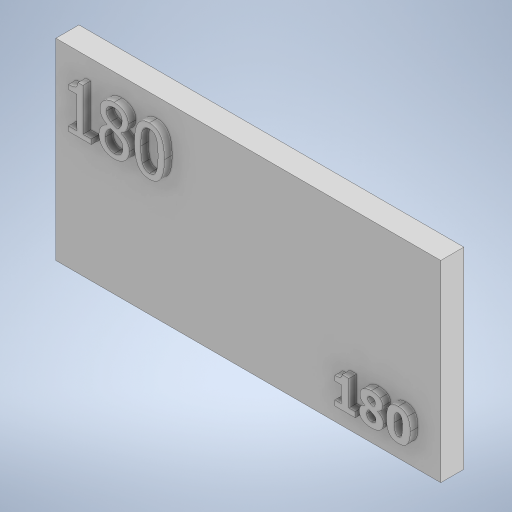
# Autodesk Inventor part: температурный тест
Saved by Autodesk Inventor 2023.1 (Build 271208000, 208)
## iProperties
Created: 2023-03-01
Part Number: температурный тест
Material: Типовые
Document SubType Name: Modeling
Designer: User
Density: 1 g/cm^3
Appearance: По умолчанию
Author: User
Autodesk Inventor part; units mm, degrees
ref_plane "YZ Plane" through (0, 0, 0) normal (1, 0, 0) x (0, 1, 0)
ref_plane "XZ Plane" through (0, 0, 0) normal (0, 1, 0) x (-1, 0, 0)
ref_plane "XY Plane" through (0, 0, 0) normal (0, 0, 1) x (1, 0, 0)
sketch "Эскиз1" plane through (0, 0, 0) normal (0, 0, 1) x (1, 0, 0)
  line L0 (-25, 12.5) -> (25, 12.5)
  line L1 (25, 12.5) -> (25, -12.5)
  line L2 (25, -12.5) -> (-25, -12.5)
  line L3 (-25, -12.5) -> (-25, 12.5)
  line L4 (0, -17.5) -> (0, 17.5) projected
  line L5 (-35, 0) -> (35, 0) projected
  line L6 (-15, 7.5) -> (15, 7.5)
  line L7 (15, 7.5) -> (15, -7.5)
  line L8 (15, -7.5) -> (-15, -7.5)
  line L9 (-15, -7.5) -> (-15, 7.5)
  point P0 (0, 0)
  dimension "d0" = 50
  dimension "d1" = 25
  dimension "d2" = 5
  dimension "d3" = 10
  constraints: 16 end point, 4 parallel, 2 horizontal, 2 perpendicular, 4 other
  measures "d0" distance between parallel lines of L1 L3
  measures "d1" distance between parallel lines of L0 L2
  measures "d2" distance between parallel lines of L0 L6
  measures "d3" distance between parallel lines of L1 L7
extrude "Выдавливание1" add sketch "Эскиз1" along normal blind 2 contours L0 L4 L6 L9 L5 L3 | L0 L1 L5 L7 L6 L4 | L5 L9 L8 L4 L2 L3 | L1 L2 L4 L8 L7 L5
sketch "Эскиз2" plane through (0, 0, 2) normal (0, 0, 1) x (1, 0, 0)
  line L0 (-25, 12.5) -> (-25, -12.5) projected
  line L1 (-25, -12.5) -> (25, -12.5) projected
  line L2 (25, -12.5) -> (25, 12.5) projected
  line L3 (25, 12.5) -> (-25, 12.5) projected
  line L4 (-15, 7.5) -> (15, 7.5) projected
  line L5 (15, 7.5) -> (15, -7.5) projected
  line L6 (15, -7.5) -> (-15, -7.5) projected
  line L7 (-15, -7.5) -> (-15, 7.5) projected
  point P0 (0, 0)
extrude "Выдавливание2" add sketch "Эскиз2" along normal blind 1 contours L3 L2 L1 L0 | L4 L5 L6 L7
sketch "Эскиз3" plane through (0, 0, 3) normal (0, 0, 1) x (1, 0, 0)
  line L0 (-23.2901, 10.0825) -> (-16.4284, 10.0825) construction
  line L1 (-16.4284, 10.0825) -> (-16.4284, 6.8962) construction
  line L2 (-16.4284, 6.8962) -> (-23.2901, 6.8962) construction
  line L3 (-23.2901, 6.8962) -> (-23.2901, 10.0825) construction
  line L4 (11.7335, -5.6604) -> (22.2456, -5.6604) construction
  line L5 (22.2456, -5.6604) -> (22.2456, -9.8451) construction
  line L6 (22.2456, -9.8451) -> (11.7335, -9.8451) construction
  line L7 (11.7335, -9.8451) -> (11.7335, -5.6604) construction
  line L8 (-19.3899, 3.8441) -> (-22.3657, 3.8441)
  line L9 (-22.3657, 3.8441) -> (-22.3657, 4.467)
  line L10 (-22.3657, 4.467) -> (-21.2584, 4.467)
  line L11 (-21.2584, 4.467) -> (-21.2584, 8.5551)
  line L12 (-21.2584, 8.5551) -> (-22.3657, 8.5551)
  line L13 (-22.3657, 8.5551) -> (-22.3657, 9.1137)
  spline S0 degree 2 poles (-22.3657, 9.1137) (-21.7379, 9.1137) (-21.1447, 9.4696) (-21.1052, 9.9639) knots 0 0 0 1 2 2 2
  line L14 (-21.1052, 9.9639) -> (-20.4724, 9.9639)
  line L15 (-20.4724, 9.9639) -> (-20.4724, 4.467)
  line L16 (-20.4724, 4.467) -> (-19.3899, 4.467)
  line L17 (-19.3899, 4.467) -> (-19.3899, 3.8441)
  spline S1 degree 2 poles (-16.4239, 3.7057) (-16.8787, 3.7057) (-17.6251, 3.9776) (-17.8871, 4.2297) knots 0 0 0 1 2 2 2
  spline S2 degree 2 poles (-17.8871, 4.2297) (-18.1441, 4.4769) (-18.4111, 5.1492) (-18.4111, 5.5298) knots 0 0 0 1 2 2 2
  spline S3 degree 2 poles (-18.4111, 5.5298) (-18.4111, 6.0241) (-17.8822, 6.8546) (-17.3779, 7.1018) knots 0 0 0 1 2 2 2
  line L18 (-17.3779, 7.1018) -> (-17.3779, 7.1265)
  spline S4 degree 2 poles (-17.3779, 7.1265) (-17.8278, 7.3885) (-18.2628, 8.0113) (-18.2628, 8.476) knots 0 0 0 1 2 2 2
  spline S5 degree 2 poles (-18.2628, 8.476) (-18.2628, 9.1631) (-17.2247, 10.0825) (-16.4239, 10.0825) knots 0 0 0 1 2 2 2
  spline S6 degree 2 poles (-16.4239, 10.0825) (-15.5934, 10.0825) (-14.5899, 9.2125) (-14.5899, 8.5304) knots 0 0 0 1 2 2 2
  spline S7 degree 2 poles (-14.5899, 8.5304) (-14.5899, 8.1201) (-15.0694, 7.3193) (-15.5193, 7.0919) knots 0 0 0 1 2 2 2
  line L19 (-15.5193, 7.0919) -> (-15.5193, 7.0672)
  spline S8 degree 2 poles (-15.5193, 7.0672) (-14.9854, 6.82) (-14.4367, 6.1082) (-14.4367, 5.5446) knots 0 0 0 1 2 2 2
  spline S9 degree 2 poles (-14.4367, 5.5446) (-14.4367, 4.7636) (-15.5736, 3.7057) (-16.4239, 3.7057) knots 0 0 0 1 2 2 2
  spline S10 degree 2 poles (-15.277, 5.4655) (-15.277, 5.8412) (-15.5736, 6.2861) (-15.9938, 6.5135) knots 0 0 0 1 2 2 2
  spline S11 degree 2 poles (-15.9938, 6.5135) (-16.1322, 6.5926) (-16.5969, 6.7755) (-16.8886, 6.8941) knots 0 0 0 1 2 2 2
  spline S12 degree 2 poles (-16.8886, 6.8941) (-17.2247, 6.6717) (-17.5856, 6.0093) (-17.5856, 5.5891) knots 0 0 0 1 2 2 2
  spline S13 degree 2 poles (-17.5856, 5.5891) (-17.5856, 5.0355) (-16.9182, 4.3137) (-16.414, 4.3137) knots 0 0 0 1 2 2 2
  spline S14 degree 2 poles (-16.414, 4.3137) (-15.8999, 4.3137) (-15.277, 4.9317) (-15.277, 5.4655) knots 0 0 0 1 2 2 2
  spline S15 degree 2 poles (-15.3907, 8.5205) (-15.3907, 8.9308) (-15.9394, 9.4795) (-16.4288, 9.4795) knots 0 0 0 1 2 2 2
  spline S16 degree 2 poles (-16.4288, 9.4795) (-16.8737, 9.4795) (-17.4422, 8.9901) (-17.4422, 8.5699) knots 0 0 0 1 2 2 2
  spline S17 degree 2 poles (-17.4422, 8.5699) (-17.4422, 8.2684) (-17.1505, 7.8482) (-16.8589, 7.6801) knots 0 0 0 1 2 2 2
  spline S18 degree 2 poles (-16.8589, 7.6801) (-16.7353, 7.6109) (-16.2113, 7.3687) (-15.9988, 7.2995) knots 0 0 0 1 2 2 2
  spline S19 degree 2 poles (-15.9988, 7.2995) (-15.6428, 7.5714) (-15.3907, 8.1497) (-15.3907, 8.5205) knots 0 0 0 1 2 2 2
  spline S20 degree 2 poles (-9.8938, 6.8941) (-9.8938, 5.253) (-10.8479, 3.7156) (-11.8415, 3.7156) knots 0 0 0 1 2 2 2
  spline S21 degree 2 poles (-11.8415, 3.7156) (-12.8499, 3.7156) (-13.7941, 5.2826) (-13.7941, 6.8892) knots 0 0 0 1 2 2 2
  spline S22 degree 2 poles (-13.7941, 6.8892) (-13.7941, 8.5402) (-12.84, 10.0677) (-11.8415, 10.0677) knots 0 0 0 1 2 2 2
  spline S23 degree 2 poles (-11.8415, 10.0677) (-10.838, 10.0677) (-9.8938, 8.4859) (-9.8938, 6.8941) knots 0 0 0 1 2 2 2
  spline S24 degree 2 poles (-10.9418, 5.0355) (-10.8232, 5.337) (-10.7243, 6.2663) (-10.7243, 6.8941) knots 0 0 0 1 2 2 2
  spline S25 degree 2 poles (-10.7243, 6.8941) (-10.7243, 7.5219) (-10.8232, 8.4463) (-10.9467, 8.7577) knots 0 0 0 1 2 2 2
  spline S26 degree 2 poles (-10.9467, 8.7577) (-11.0703, 9.0692) (-11.5004, 9.3905) (-11.8415, 9.3905) knots 0 0 0 1 2 2 2
  spline S27 degree 2 poles (-11.8415, 9.3905) (-12.1826, 9.3905) (-12.6225, 9.0692) (-12.751, 8.7479) knots 0 0 0 1 2 2 2
  spline S28 degree 2 poles (-12.751, 8.7479) (-12.8746, 8.4364) (-12.9636, 7.4873) (-12.9636, 6.8892) knots 0 0 0 1 2 2 2
  spline S29 degree 2 poles (-12.9636, 6.8892) (-12.9636, 6.2466) (-12.8845, 5.3864) (-12.756, 5.0503) knots 0 0 0 1 2 2 2
  spline S30 degree 2 poles (-12.756, 5.0503) (-12.6373, 4.7339) (-12.1974, 4.3928) (-11.8415, 4.3928) knots 0 0 0 1 2 2 2
  spline S31 degree 2 poles (-11.8415, 4.3928) (-11.5053, 4.3928) (-11.0654, 4.7142) (-10.9418, 5.0355) knots 0 0 0 1 2 2 2
  line L20 (14.9004, -9.7511) -> (12.2586, -9.7511)
  line L21 (12.2586, -9.7511) -> (12.2586, -9.0542)
  line L22 (12.2586, -9.0542) -> (13.1014, -9.0542)
  line L23 (13.1014, -9.0542) -> (13.1014, -6.9375)
  line L24 (13.1014, -6.9375) -> (12.2586, -6.9375)
  line L25 (12.2586, -6.9375) -> (12.2586, -6.286)
  spline S32 degree 2 poles (12.2586, -6.286) (12.4434, -6.286) (12.8097, -6.2374) (12.9199, -6.1855) knots 0 0 0 1 2 2 2
  spline S33 degree 2 poles (12.9199, -6.1855) (13.0463, -6.1207) (13.1889, -5.9035) (13.2019, -5.7414) knots 0 0 0 1 2 2 2
  line L26 (13.2019, -5.7414) -> (14.0771, -5.7414)
  line L27 (14.0771, -5.7414) -> (14.0771, -9.0542)
  line L28 (14.0771, -9.0542) -> (14.9004, -9.0542)
  line L29 (14.9004, -9.0542) -> (14.9004, -9.7511)
  spline S34 degree 2 poles (18.573, -8.6393) (18.573, -8.8954) (18.3591, -9.3395) (18.1549, -9.5015) knots 0 0 0 1 2 2 2
  spline S35 degree 2 poles (18.1549, -9.5015) (17.9507, -9.6636) (17.364, -9.8451) (16.9847, -9.8451) knots 0 0 0 1 2 2 2
  spline S36 degree 2 poles (16.9847, -9.8451) (16.5795, -9.8451) (15.9734, -9.6604) (15.7789, -9.5015) knots 0 0 0 1 2 2 2
  spline S37 degree 2 poles (15.7789, -9.5015) (15.5876, -9.3427) (15.4061, -8.9116) (15.4061, -8.6717) knots 0 0 0 1 2 2 2
  spline S38 degree 2 poles (15.4061, -8.6717) (15.4061, -8.3281) (15.7854, -7.8711) (16.1452, -7.7187) knots 0 0 0 1 2 2 2
  line L30 (16.1452, -7.7187) -> (16.1452, -7.7025)
  spline S39 degree 2 poles (16.1452, -7.7025) (15.7918, -7.5307) (15.5131, -7.0413) (15.5131, -6.7398) knots 0 0 0 1 2 2 2
  spline S40 degree 2 poles (15.5131, -6.7398) (15.5131, -6.5194) (15.7076, -6.1336) (15.8988, -5.9813) knots 0 0 0 1 2 2 2
  spline S41 degree 2 poles (15.8988, -5.9813) (16.0836, -5.8354) (16.6443, -5.6604) (16.9944, -5.6604) knots 0 0 0 1 2 2 2
  spline S42 degree 2 poles (16.9944, -5.6604) (17.364, -5.6604) (17.915, -5.8192) (18.0933, -5.9489) knots 0 0 0 1 2 2 2
  spline S43 degree 2 poles (18.0933, -5.9489) (18.2748, -6.0785) (18.4693, -6.4545) (18.4693, -6.6717) knots 0 0 0 1 2 2 2
  spline S44 degree 2 poles (18.4693, -6.6717) (18.4693, -6.957) (18.1387, -7.414) (17.7983, -7.5729) knots 0 0 0 1 2 2 2
  line L31 (17.7983, -7.5729) -> (17.7983, -7.5858)
  spline S45 degree 2 poles (17.7983, -7.5858) (18.197, -7.7479) (18.573, -8.273) (18.573, -8.6393) knots 0 0 0 1 2 2 2
  spline S46 degree 2 poles (17.5811, -8.6814) (17.5811, -8.4837) (17.4126, -8.2763) (17.1403, -8.1434) knots 0 0 0 1 2 2 2
  spline S47 degree 2 poles (17.1403, -8.1434) (17.0625, -8.1077) (16.7675, -7.9943) (16.6541, -7.9456) knots 0 0 0 1 2 2 2
  spline S48 degree 2 poles (16.6541, -7.9456) (16.5503, -8.0494) (16.385, -8.3605) (16.385, -8.5453) knots 0 0 0 1 2 2 2
  spline S49 degree 2 poles (16.385, -8.5453) (16.385, -8.8241) (16.7416, -9.1579) (17.0301, -9.1579) knots 0 0 0 1 2 2 2
  spline S50 degree 2 poles (17.0301, -9.1579) (17.1111, -9.1579) (17.3121, -9.1061) (17.3899, -9.0542) knots 0 0 0 1 2 2 2
  spline S51 degree 2 poles (17.3899, -9.0542) (17.4774, -8.9926) (17.5811, -8.8241) (17.5811, -8.6814) knots 0 0 0 1 2 2 2
  spline S52 degree 2 poles (17.4936, -6.7884) (17.4936, -6.5842) (17.2246, -6.3411) (16.9944, -6.3411) knots 0 0 0 1 2 2 2
  spline S53 degree 2 poles (16.9944, -6.3411) (16.774, -6.3411) (16.505, -6.5615) (16.505, -6.7236) knots 0 0 0 1 2 2 2
  spline S54 degree 2 poles (16.505, -6.7236) (16.505, -6.8824) (16.667, -7.0802) (16.8388, -7.1612) knots 0 0 0 1 2 2 2
  spline S55 degree 2 poles (16.8388, -7.1612) (16.9134, -7.2001) (17.1208, -7.2811) (17.2926, -7.346) knots 0 0 0 1 2 2 2
  spline S56 degree 2 poles (17.2926, -7.346) (17.3964, -7.2098) (17.4936, -6.9537) (17.4936, -6.7884) knots 0 0 0 1 2 2 2
  spline S57 degree 2 poles (22.0349, -7.7511) (22.0349, -8.2698) (21.8696, -9.0477) (21.6849, -9.3103) knots 0 0 0 1 2 2 2
  spline S58 degree 2 poles (21.6849, -9.3103) (21.5033, -9.5696) (20.9166, -9.8354) (20.4952, -9.8354) knots 0 0 0 1 2 2 2
  spline S59 degree 2 poles (20.4952, -9.8354) (20.0706, -9.8354) (19.4871, -9.5696) (19.3024, -9.3038) knots 0 0 0 1 2 2 2
  spline S60 degree 2 poles (19.3024, -9.3038) (19.1176, -9.0413) (18.9523, -8.2698) (18.9523, -7.7511) knots 0 0 0 1 2 2 2
  spline S61 degree 2 poles (18.9523, -7.7511) (18.9523, -7.2195) (19.1176, -6.4675) (19.3056, -6.1952) knots 0 0 0 1 2 2 2
  spline S62 degree 2 poles (19.3056, -6.1952) (19.4936, -5.9294) (20.0868, -5.6701) (20.4952, -5.6701) knots 0 0 0 1 2 2 2
  spline S63 degree 2 poles (20.4952, -5.6701) (20.9264, -5.6701) (21.5033, -5.9424) (21.6881, -6.2114) knots 0 0 0 1 2 2 2
  spline S64 degree 2 poles (21.6881, -6.2114) (21.8696, -6.474) (22.0349, -7.2487) (22.0349, -7.7511) knots 0 0 0 1 2 2 2
  spline S65 degree 2 poles (21.0268, -7.7511) (21.0268, -7.0088) (20.7837, -6.4092) (20.4952, -6.4092) knots 0 0 0 1 2 2 2
  spline S66 degree 2 poles (20.4952, -6.4092) (20.2067, -6.4092) (19.9604, -7.0088) (19.9604, -7.7544) knots 0 0 0 1 2 2 2
  spline S67 degree 2 poles (19.9604, -7.7544) (19.9604, -8.487) (20.2067, -9.0964) (20.4952, -9.0964) knots 0 0 0 1 2 2 2
  spline S68 degree 2 poles (20.4952, -9.0964) (20.7805, -9.0964) (21.0268, -8.487) (21.0268, -7.7511) knots 0 0 0 1 2 2 2
  point P0 (0, 0)
  constraints: 4 other
extrude "Выдавливание3" add sketch "Эскиз3" along normal blind 1
